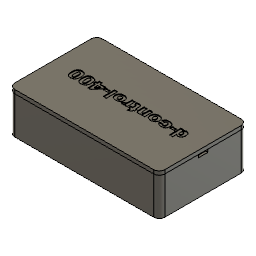
d-control-400-remote-enclosure (Autodesk Fusion 360 design; units mm, degrees)
part number: 2026-07-07-16-35-03-967
Autodesk Fusion 360 part; units mm, degrees
note: some values were not read from the file. Set by a fixed rule: which face or edge a step refers to.
sketch "case" plane through (0, 0, 0) normal (0, 1, 0) x (1, 0, 0)
  line L0 (0, 0) -> (80, 0)
  line L1 (80, 0) -> (80, -46.7)
  line L2 (80, -46.7) -> (0, -46.7)
  line L3 (0, -46.7) -> (0, 0)
  dimension "d1" = 80
  dimension "d2" = 46.7
  constraint horizontal L0
  constraint vertical L1
  constraint horizontal L2
  constraint vertical L3
  constraint coincident L0.start L3.end
  measures "d1" distance of L0.start L0.end
  measures "d2" distance of L0.start L2.end
extrude "Extrude1" add sketch "case" along normal blind 20 makes body 1
shell "Shell1" thickness 2 removed faces 1 at (26.6667, 20, 15.5667) on bodies 1
sketch "standoff" plane through (0, 2, 0) normal (0, 1, 0) x (-1, 0, 0)
  circle A0 centre (-8.85, 41.95) radius 2.75
  line L0 (-78, 2) -> (-2, 2)
  line L1 (-2, 45) -> (-78, 45)
  line L2 (-2, 2) -> (-2, 45)
  line L3 (-2, 45) -> (-78, 45)
  line L4 (-78, 45) -> (-78, 2)
  line L5 (-78, 2) -> (-2, 2)
  line L6 (-2, 44.7) -> (-78, 44.7)
  line L7 (-78, 44.7) -> (-78, 2)
  line L8 (-78, 2) -> (-2, 2)
  line L9 (-2, 2) -> (-2, 44.7)
  dimension "d42" = 5.5
  dimension "d59" = 6.85
  constraint tangent A0 L6
  measures "d42" diameter of A0
  measures "d59" distance of A0.centre L2
extrude "Extrude7" add sketch "standoff" along normal blind 5 contours A0 bodies 1
sketch "standoff_hole" plane through (0, 7, 0) normal (0, 1, 0) x (-1, 0, 0)
  circle A0 centre (-8.85, 41.95) radius 0.9
  circle A1 centre (-8.85, 41.95) radius 2.75
  circle A2 centre (-8.85, 41.95) radius 2.75
  dimension "d47" = 1.8
  constraint concentric A0 A1
  measures "d47" diameter of A0
extrude "Extrude8" cut sketch "standoff_hole" against normal blind 4 contours A0 bodies 1
pattern_linear "R-Pattern3" count 2 spacing 37.2 along (0, 0, -1) of "Extrude7", "Extrude8"
pattern_linear "R-Pattern4" count 2 spacing 45 along (1, 0, 0) of "Extrude7", "Extrude8", "R-Pattern3"
sketch "usb-c_hole" plane through (0, 0, 0) normal (-1, 0, 0) x (0, 0, 1)
  line L0 (0, 0) -> (46.7, 0)
  line L1 (46.7, 0) -> (46.7, 20)
  line L2 (46.7, 20) -> (0, 20)
  line L3 (0, 20) -> (0, 0)
  line L4 (23.35, 20) -> (23.35, 0) construction
  line L5 (20.4338, 9.5) -> (26.2662, 9.5)
  arc A0 (26.2662, 9.5) -> (26.2662, 16.5) centre (26.2662, 13) ccw
  line L6 (26.2662, 16.5) -> (20.4338, 16.5)
  arc A1 (20.4338, 16.5) -> (20.4338, 9.5) centre (20.4338, 13) ccw
  line L7 (20.4338, 13) -> (26.2662, 13) construction
  point P0 (23.35, 13)
  point P1 (16.9338, 13)
  point P2 (29.7662, 13)
  dimension "d63" = 7
  dimension "d64" = 13
  constraint midpoint L2 L4.start
  constraint midpoint L0 L4.end
  constraint tangent L5 A0
  constraint tangent A0 L6
  constraint parallel L5 L6
  constraint tangent L6 A1
  constraint tangent L5 A1
  constraint perpendicular L4 L7
  constraint midpoint L7 P0
  constraint coincident L4 P0
  constraint midpoint A1 P1
  constraint midpoint A0 P2
  measures "d63" diameter of A0
  measures "d64" distance of L0 P0
extrude "Extrude9" cut sketch "usb-c_hole" against normal up to surface (2 mm away) contours L5 A0 L6 A1 bodies 1
sketch "lid" plane through (0, 20, 0) normal (0, 1, 0) x (-1, 0, 0)
  line L0 (-2, 44.7) -> (-2, 2)
  line L1 (-2, 2) -> (-78, 2)
  line L2 (-78, 2) -> (-78, 44.7)
  line L3 (-78, 44.7) -> (-2, 44.7)
  line L4 (0, 46.7) -> (-80, 46.7)
  line L5 (-80, 46.7) -> (-80, 0)
  line L6 (-80, 0) -> (0, 0)
  line L7 (0, 0) -> (0, 46.7)
  line L8 (-80, 46.7) -> (0, 46.7)
  line L9 (0, 46.7) -> (0, 0)
  line L10 (0, 0) -> (-80, 0)
  line L11 (-80, 0) -> (-80, 46.7)
  line L12 (0, 0) -> (0, 46.7)
extrude "Extrude10" add sketch "lid" along normal blind 2 separate body contours L0 L1 L2 L3 | L4 L5 L6 L7 L8 L9 L10 L11 L12 makes body 2
extrude "Extrude11" add sketch "lid" against normal blind 3 contours L0 L1 L2 L3 bodies 2
move_face "OffsetFaces1" offset -0.1 4 faces at (78, 19, 16.2333) (27.3333, 18, 2) (2, 19, 30.4667) (52.6667, 18, 44.7) on bodies 2
chamfer "Chamfer1" distance 0.5 angle 45 4 edges at (40, 17, 44.6) (77.9, 17, 23.35) (40, 17, 2.1) (2.1, 17, 23.35) tangent chain off on bodies 2
sketch "lid_text" plane through (0, 22, 0) normal (0, 1, 0) x (-1, 0, 0)
  line L0 (-80, 0) -> (0, 0)
  line L1 (0, 0) -> (0, 46.7)
  line L2 (0, 46.7) -> (-80, 46.7)
  line L3 (-80, 46.7) -> (-80, 0)
  line L4 (-80, 0) -> (0, 0) construction
  line L5 (0, 0) -> (0, 46.7) construction
  line L6 (0, 46.7) -> (-80, 46.7) construction
  line L7 (-80, 46.7) -> (-80, 0) construction
  dimension "d73" = 6
  dimension "d74" = 0
  text T0 "d-control-400" font "Arial Black" height 6 align centre middle in box 80 x 46.7 at (-80, 0) x (1, 0) y (0, 1) spacing 1
  constraint coincident L0.end
  constraint coincident L2.end
extrude "Extrude12" cut sketch "lid_text" against normal blind 0.4 text T0 bodies 2
sketch "pry_notch" plane through (80, 0, 0) normal (1, 0, 0) x (0, 0, -1)
  line L0 (-46.7, 0) -> (0, 0)
  line L1 (0, 0) -> (0, 20)
  line L2 (0, 20) -> (-46.7, 20)
  line L3 (-46.7, 20) -> (-46.7, 0)
  line L4 (-25.85, 20) -> (-20.85, 20)
  line L5 (-20.85, 20) -> (-20.85, 18.5)
  line L6 (-20.85, 18.5) -> (-25.85, 18.5)
  line L7 (-25.85, 18.5) -> (-25.85, 20)
  dimension "d77" = 5
  dimension "d78" = 1.5
  constraint horizontal L4
  constraint vertical L5
  constraint horizontal L6
  constraint vertical L7
  constraint midpoint L2 L4
  measures "d77" distance of L4.start L4.end
  measures "d78" distance of L4.start L6.end
extrude "Extrude13" cut sketch "pry_notch" against normal blind 1.2 contours L2 L4 L5 L6 L7 bodies 1
fillet "Fillet1" radius 3 4 edges at (80, 10, 0) (80, 10, 46.7) (0, 10, 46.7) (0, 10, 0) on bodies 1
fillet "Fillet2" radius 3 4 edges at (0, 21, 0) (0, 21, 46.7) (80, 21, 0) (80, 21, 46.7) on bodies 2
equation "d74 = 'd-control-400'"
named bodies: "case", "lid"
